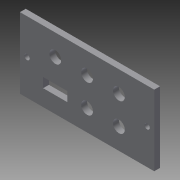
# Autodesk Inventor part: 5 led cap
Saved by Autodesk Inventor 2014 SP1 (Build 180222100, 222)
## iProperties
Created: 2017-07-20
Part Number: 5 led cap
Material: Generic
Document SubType Name: Modeling
Designer: kteo17
Density: 1 g/cm^3
Appearance: Default
Author: kteo17
Autodesk Inventor part; units mm, degrees
ref_plane "YZ Plane" through (0, 0, 0) normal (1, 0, 0) x (0, 1, 0)
ref_plane "XZ Plane" through (0, 0, 0) normal (0, 1, 0) x (-1, 0, 0)
ref_plane "XY Plane" through (0, 0, 0) normal (0, 0, 1) x (1, 0, 0)
sketch "Sketch1" plane through (0, 0, 0) normal (0, 0, 1) x (1, 0, 0)
  line L0 (0, 0) -> (60.325, 0)
  line L1 (60.325, 0) -> (60.325, 31.75)
  line L2 (60.325, 31.75) -> (0, 31.75)
  line L3 (0, 31.75) -> (0, 0)
  circle A0 centre (3.175, 15.875) radius 1.1938
  circle A1 centre (57.15, 15.875) radius 1.1938
  line L4 (21.336, 11.684) -> (10.414, 11.684)
  line L5 (10.414, 11.684) -> (10.414, 7.366)
  line L6 (10.414, 7.366) -> (21.336, 7.366)
  line L7 (21.336, 7.366) -> (21.336, 11.684)
  line L8 (21.336, 11.684) -> (10.414, 7.366) construction
  line L9 (10.414, 11.684) -> (21.336, 7.366) construction
  circle A2 centre (15.875, 22.225) radius 2.667
  circle A3 centre (30.1625, 22.225) radius 2.667
  circle A4 centre (44.45, 22.225) radius 2.667
  circle A5 centre (30.1625, 9.525) radius 2.667
  circle A6 centre (44.45, 9.525) radius 2.667
  point P0 (15.875, 9.525)
  dimension "d0" = 60.325
  dimension "d1" = 31.75
  dimension "d2" = 2.3876
  dimension "d3" = 2.3876
  dimension "d4" = 10.922
  dimension "d5" = 4.318
  dimension "d6" = 5.334
  dimension "d7" = 5.334
  dimension "d8" = 5.334
  dimension "d9" = 5.334
  dimension "d10" = 5.334
  constraints: 20 end point, 7 centre point, 4 parallel, 2 horizontal, 2 midpoint, 2 perpendicular
  measures "d0" distance of L2.end L1.end
  measures "d1" distance of L1.end L0.end
  measures "d2" diameter of A0
  measures "d3" diameter of A1
  measures "d4" distance of L6.end L5.end
  measures "d5" distance of L5.end L4.end
  measures "d6" diameter of A2
  measures "d7" diameter of A3
  measures "d8" diameter of A4
  measures "d9" diameter of A5
  measures "d10" diameter of A6
extrude "Extrusion1" add sketch "Sketch1" along normal blind 2.6162
body "Solid1"
